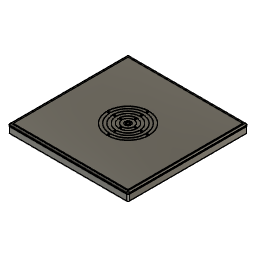
case (Autodesk Fusion 360 design; units mm, degrees)
Autodesk Fusion 360 part; units mm, degrees
sketch "Sketch1" plane through (0, 0, 0) normal (0, 0, 1) x (1, 0, 0)
  line L0 (50, 50) -> (-50, 50)
  line L1 (-50, 50) -> (-50, -50)
  line L2 (-50, -50) -> (50, -50)
  line L3 (50, -50) -> (50, 50)
  line L4 (50, 50) -> (-50, -50) construction
  line L5 (-50, 50) -> (50, -50) construction
  dimension "d1" = 100
  dimension "d2" = 100
  constraint horizontal L0
  constraint perpendicular L0 L1
  constraint parallel L0 L2
  constraint parallel L1 L3
  constraint coincident L4 origin
  constraint coincident L5 origin
  measures "d1" distance of L1.end L2.end
  measures "d2" distance of L0 L2
extrude "Extrude1" add sketch "Sketch1" along normal blind 7 makes body 1
ref_plane "WorkPlane1" through (0, 0, 5) normal (0, 0, -1) x (-1, 0, 0)
split "Split1" by plane through (0, 0, 5) normal (0, 0, -1) bodies 1 makes body 2 at (-16.6667, 16.6667, 0)
shell "Shell1" thickness 2 removed faces 0 bodies 2
sketch "Sketch3" plane through (0, 0, 5) normal (0, 0, 1) x (-1, 0, 0)
  line L0 (50, 50) -> (-50, 50)
  line L1 (-50, 50) -> (-50, -50)
  line L2 (-50, -50) -> (50, -50)
  line L3 (50, -50) -> (50, 50)
  line L4 (48, -48) -> (-48, -48)
  line L5 (-48, -48) -> (-48, 48)
  line L6 (-48, 48) -> (48, 48)
  line L7 (48, 48) -> (48, -48)
  dimension "d7" = 2
  dimension "d8" = 2
  dimension "d9" = 2
  dimension "d10" = 2
  constraint horizontal L4
  constraint vertical L5
  constraint horizontal L6
  constraint vertical L7
  measures "d7" distance of L2 L4
  measures "d8" distance of L3 L7
  measures "d9" distance of L0 L6
  measures "d10" distance of L1 L5
extrude "Extrude2" cut sketch "Sketch3" against normal blind 4.7 contours L4 L5 L6 L7 bodies 2
sketch "Sketch4" plane through (0, 0, 0) normal (0, 0, 1) x (1, 0, 0)
  line L0 (-48, 48) -> (48, 48)
  line L1 (48, 48) -> (48, -48)
  line L2 (48, -48) -> (-48, -48)
  line L3 (-48, -48) -> (-48, 48)
  line L4 (-50, -50) -> (-50, 50)
  line L5 (50, -50) -> (-50, -50)
  line L6 (50, 50) -> (50, -50)
  line L7 (-50, 50) -> (50, 50)
  dimension "d13" = 2
  dimension "d14" = 2
  dimension "d15" = 2
  dimension "d16" = 2
  constraint horizontal L0
  constraint vertical L1
  constraint horizontal L2
  constraint vertical L3
  measures "d13" distance of L3 L4
  measures "d14" distance of L2 L5
  measures "d15" distance of L1 L6
  measures "d16" distance of L0 L7
extrude "Extrude3" cut sketch "Sketch4" along normal blind 6.8 contours L0 L1 L2 L3 bodies 1
fillet "Fillet1" radius 1 2 edges at (50, -50, 6) (50, -50, 2.5) on bodies 1 2
fillet "Fillet2" radius 1 2 edges at (50, 50, 6) (50, 50, 2.5) on bodies 1 2
fillet "Fillet3" radius 1 2 edges at (-50, 50, 6) (-50, 50, 2.5) on bodies 1 2
fillet "Fillet4" radius 1 2 edges at (-50, -50, 6) (-50, -50, 2.5) on bodies 1 2
fillet "Fillet5" radius 1 8 edges at (-49.7071, -49.7071, 7) (0, -50, 7) (49.7071, -49.7071, 7) (50, 0, 7) (49.7071, 49.7071, 7) (0, 50, 7) (-49.7071, 49.7071, 7) (-50, 0, 7) on bodies 1
sketch "Sketch5" plane through (0, 0, 7) normal (0, 0, 1) x (-1, 0, 0)
  line L0 (49, 49) -> (-49, 49)
  line L1 (-49, 49) -> (-49, -49)
  line L2 (-49, -49) -> (49, -49)
  line L3 (49, -49) -> (49, 49)
  circle A0 centre (0, 0) radius 2.5
  line L4 (0.5, -20.5) -> (0.5, 20.5)
  line L5 (-0.5, 20.5) -> (-0.5, -20.5)
  line L6 (20.5, 0.5) -> (-20.5, 0.5)
  line L7 (-20.5, -0.5) -> (20.5, -0.5)
  arc A1 (4.9749, 0.5) -> (0.5, 4.9749) centre (0, 0) ccw
  arc A2 (7.4833, 0.5) -> (0.5, 7.4833) centre (0, 0) ccw
  arc A3 (9.9875, 0.5) -> (0.5, 9.9875) centre (0, 0) ccw
  arc A4 (12.49, 0.5) -> (0.5, 12.49) centre (0, 0) ccw
  arc A5 (14.9917, 0.5) -> (0.5, 14.9917) centre (0, 0) ccw
  arc A6 (17.4929, 0.5) -> (0.5, 17.4929) centre (0, 0) ccw
  arc A7 (19.9937, 0.5) -> (0.5, 19.9937) centre (0, 0) ccw
  arc A8 (0.5, -19.9937) -> (19.9937, -0.5) centre (0, 0) ccw
  arc A9 (0.5, -17.4929) -> (17.4929, -0.5) centre (0, 0) ccw
  arc A10 (0.5, -14.9917) -> (14.9917, -0.5) centre (0, 0) ccw
  arc A11 (0.5, -12.49) -> (12.49, -0.5) centre (0, 0) ccw
  arc A12 (0.5, -9.9875) -> (9.9875, -0.5) centre (0, 0) ccw
  arc A13 (0.5, -7.4833) -> (7.4833, -0.5) centre (0, 0) ccw
  arc A14 (0.5, -4.9749) -> (4.9749, -0.5) centre (0, 0) ccw
  arc A15 (-0.5, 19.9937) -> (-19.9937, 0.5) centre (0, 0) ccw
  arc A16 (-19.9937, -0.5) -> (-0.5, -19.9937) centre (0, 0) ccw
  arc A17 (-0.5, 17.4929) -> (-17.4929, 0.5) centre (0, 0) ccw
  arc A18 (-17.4929, -0.5) -> (-0.5, -17.4929) centre (0, 0) ccw
  arc A19 (-0.5, 14.9917) -> (-14.9917, 0.5) centre (0, 0) ccw
  arc A20 (-14.9917, -0.5) -> (-0.5, -14.9917) centre (0, 0) ccw
  arc A21 (-0.5, 12.49) -> (-12.49, 0.5) centre (0, 0) ccw
  arc A22 (-12.49, -0.5) -> (-0.5, -12.49) centre (0, 0) ccw
  arc A23 (-0.5, 9.9875) -> (-9.9875, 0.5) centre (0, 0) ccw
  arc A24 (-9.9875, -0.5) -> (-0.5, -9.9875) centre (0, 0) ccw
  arc A25 (-0.5, 7.4833) -> (-7.4833, 0.5) centre (0, 0) ccw
  arc A26 (-7.4833, -0.5) -> (-0.5, -7.4833) centre (0, 0) ccw
  arc A27 (-0.5, 4.9749) -> (-4.9749, 0.5) centre (0, 0) ccw
  arc A28 (-4.9749, -0.5) -> (-0.5, -4.9749) centre (0, 0) ccw
  dimension "d29" = 5
  dimension "d30" = 10
  dimension "d31" = 15
  dimension "d32" = 20
  dimension "d33" = 25
  dimension "d34" = 30
  dimension "d35" = 35
  dimension "d36" = 40
  constraint coincident A0.centre A1.centre
  constraint concentric A0 A27
  constraint concentric A0 A25
  constraint concentric A0 A21
  constraint concentric A19 A23
  constraint concentric A15 A23
  constraint vertical L4
  constraint vertical L5
  constraint horizontal L6
  constraint horizontal L7
  constraint coincident L4 A7.end
  constraint coincident L5 A15.start
  constraint coincident L4 A6.end
  constraint coincident L5 A17.start
  constraint coincident L4 A5.end
  constraint coincident L5 A19.start
  constraint coincident L4 A4.end
  constraint coincident L5 A21.start
  constraint coincident L4 A3.end
  constraint coincident L5 A23.start
  constraint coincident L4 A2.end
  constraint coincident L5 A25.start
  constraint coincident L4 A1.end
  constraint coincident L5 A27.start
  constraint coincident L7 A14.end
  constraint coincident L6 A1.start
  constraint concentric A1 A27
  constraint coincident L7 A13.end
  constraint coincident L6 A2.start
  constraint concentric A2 A25
  constraint coincident L7 A12.end
  constraint coincident L6 A3.start
  constraint concentric A3 A23
  constraint coincident L7 A11.end
  constraint coincident L6 A4.start
  constraint concentric A4 A21
  constraint coincident L7 A10.end
  constraint coincident L6 A5.start
  constraint concentric A5 A19
  constraint coincident L7 A9.end
  constraint coincident L6 A6.start
  constraint concentric A6 A17
  constraint coincident L7 A8.end
  constraint coincident L6 A7.start
  constraint concentric A7 A15
  constraint coincident L5 A16.end
  constraint coincident L4 A8.start
  constraint concentric A8 A15
  constraint coincident L5 A18.end
  constraint coincident L4 A9.start
  constraint concentric A9 A17
  constraint coincident L5 A20.end
  constraint coincident L4 A10.start
  constraint concentric A10 A19
  constraint coincident L5 A22.end
  constraint coincident L4 A11.start
  constraint concentric A11 A21
  constraint coincident L5 A24.end
  constraint coincident L4 A12.start
  constraint concentric A12 A23
  constraint coincident L5 A26.end
  constraint coincident L4 A13.start
  constraint concentric A13 A25
  constraint coincident L5 A28.end
  constraint coincident L4 A14.start
  constraint concentric A14 A27
  constraint coincident L6 A15.end
  constraint coincident L7 A16.start
  constraint concentric A15 A16
  constraint coincident L6 A17.end
  constraint coincident L7 A18.start
  constraint concentric A17 A18
  constraint coincident L6 A19.end
  constraint coincident L7 A20.start
  constraint concentric A19 A20
  constraint coincident L6 A21.end
  constraint coincident L7 A22.start
  constraint concentric A21 A22
  constraint coincident L6 A23.end
  constraint coincident L7 A24.start
  constraint concentric A23 A24
  constraint coincident L6 A25.end
  constraint coincident L7 A26.start
  constraint concentric A25 A26
  constraint coincident L6 A27.end
  constraint coincident L7 A28.start
  constraint concentric A27 A28
  measures "d29" diameter of A0
  measures "d30" diameter of A27
  measures "d31" diameter of A25
  measures "d32" diameter of A23
  measures "d33" diameter of A21
  measures "d34" diameter of A19
  measures "d35" diameter of A17
  measures "d36" diameter of A15
extrude "Extrude4" cut sketch "Sketch5" along normal blind 10 and the other way through all contours A0 L4 L6 | A0 L4 L7 | L4 L6 A1 A2 | L4 L7 A13 A14 | A0 L5 L6 | A0 L5 L7 | L5 L6 A25 A27 | L4 L6 A3 A4 | L5 L7 A26 A28 | L4 L7 A11 A12 | L5 L6 A21 A23 | L4 L6 A5 A6 | L5 L7 A22 A24 | L4 L7 A9 A10 | L5 L6 A17 A19 | L5 L7 A18 A20 bodies 1
named bodies: "Tampa", "Base"
